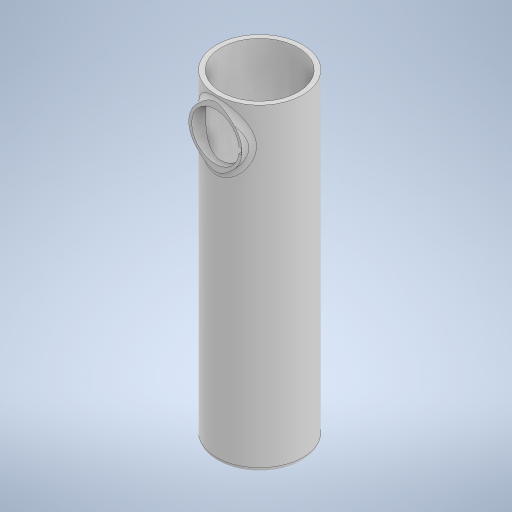
# Autodesk Inventor part: Flash_light
Saved by Autodesk Inventor 2024.2 (Build 282272000, 272)
## iProperties
Created: 2025-04-08
Part Number: Flash_light
Material: Generic
Document SubType Name: Modeling
Designer: Svend
Density: 1 g/cm^3
Appearance: Default
Author: Svend
Autodesk Inventor part; units mm, degrees
ref_plane "YZ Plane" through (0, 0, 0) normal (1, 0, 0) x (0, 1, 0)
sketch "Sketch1" plane through (0, 0, 0) normal (0, 1, 0) x (-1, 0, 0)
  circle A0 centre (0, 0) radius 15
  circle A1 centre (0, 0) radius 18.2
  dimension "d0" = 30
  dimension "d1" = 36.4
  constraints: 2 centre point, 2 coincident
  measures "d0" diameter of A0
  measures "d1" diameter of A1
extrude "Extrusion1" add sketch "Sketch1" along normal blind 4 contours A0 | A1
sketch "Sketch2" plane through (0, 4, 0) normal (0, -1, 0) x (1, 0, 0)
  circle A0 centre (0, 0) radius 18.2 projected
  circle A1 centre (0, 0) radius 16.2
  dimension "d17" = 2
  constraints: 1 centre point
  measures "d17" radial gap between concentric circles of A0 A1
extrude "Extrusion2" add sketch "Sketch2" against normal blind 130
ref_plane "Work Plane1" through (0, 0, 18.6) normal (0, 0, 1) x (1, 0, 0)
ref_plane "Work Plane2" through (0, 0, 18.2) normal (0, 0, 1) x (1, 0, 0)
sketch "Sketch3" plane through (0, 0, 18.6) normal (0, 0, 1) x (1, 0, 0)
  line L0 (0, 134) -> (0, 119) construction
  circle A0 centre (0, 119) radius 10
  circle A1 centre (0, 119) radius 11.2
  line L1 (11, 120.2) -> (9.9277, 120.2)
  line L2 (9, 120.2) -> (9, 117.8) construction
  line L3 (9, 117.8) -> (9.9277, 117.8) construction
  line L4 (11, 117.8) -> (11, 120.2)
  line L5 (11, 120.2) -> (9, 117.8) construction
  line L6 (9, 120.2) -> (11, 117.8) construction
  line L7 (9.9277, 120.2) -> (9, 120.2) construction
  line L8 (9.9277, 117.8) -> (11, 117.8)
  line L9 (18.2, 134) -> (-18.2, 134) projected
  line L10 (0, 134) -> (0, 119) construction
  point P0 (0, 0)
  point P1 (10, 119)
  dimension "d9" = 20
  dimension "d19" = 1.2
  dimension "d29" = 1
  dimension "d30" = 2.4
  dimension "d31" = 15
  constraints: 20 end point, 5 parallel, 3 midpoint, 3 point on circle, 2 centre point, 2 horizontal, 2 perpendicular, 2 vertical, 1 coincident, 1 horizontal alignment, 1 vertical alignment
  measures "d9" diameter of A0
  measures "d19" radial gap between concentric circles of A1 A0
  measures "d29" distance from line of L4 A0.start
  measures "d30" distance of L4.start L1.start
  measures "d31" distance of L10.start L0.end
extrude "Extrusion4" add sketch "Sketch3" against normal up to surface contours A0 | A0 L1 L4 L8 | A1 round surface about axis through (0, 0, 0) along (0, 1, 0) radius 18.2 far side no
extrude "Extrusion3" cut sketch "Sketch3" against normal blind 10 contours A0 | A0 L1 L4 L8
fillet "Fillet1" radius 3 3 edges at (8.5118, 111.7206, 16.0869) (8.5097, 126.2819, 16.0881) (-11.2, 118.9944, 14.3457)
fillet "Fillet2" radius 2 1 edges at (18.2, 0, 0)
ref_plane "Work Plane3" through (0, 0, 17.6) normal (0, 0, 1) x (1, 0, 0)
sketch "Sketch4" plane through (0, 0, 17.6) normal (0, 0, 1) x (1, 0, 0)
  line L0 (-4.6347, 132.1337) -> (-4.6347, 134) projected
  line L1 (-4.6347, 134) -> (4.6347, 134) projected
  line L2 (4.6347, 134) -> (4.6347, 132.1337) projected
  arc A0 (9.3217, 112.7915) -> (9.3217, 125.2085) centre (0, 119) ccw projected
  line L3 (4.6347, 105.8663) -> (4.6347, 2) projected
  line L4 (-4.6347, 2) -> (-4.6347, 105.8663) projected
  arc A1 (-9.3217, 125.2085) -> (-9.3217, 112.7915) centre (0, 119) ccw projected
  line L5 (0, 89) -> (-10, 89) construction
  line L6 (0, 89) -> (10, 89) construction
  line L7 (-2.5, 78) -> (2.5, 78)
  line L8 (2.5, 78) -> (2.5, 100)
  line L9 (2.5, 100) -> (-2.5, 100)
  line L10 (-2.5, 100) -> (-2.5, 78)
  line L11 (-2.5, 78) -> (2.5, 100) construction
  line L12 (2.5, 78) -> (-2.5, 100) construction
  line L13 (11, 120.2) -> (9.9277, 120.2) projected
  arc A2 (9.9277, 120.2) -> (9.9277, 117.8) centre (0, 119) ccw projected
  line L14 (9.9277, 117.8) -> (11, 117.8) projected
  line L15 (11, 117.8) -> (11, 120.2) projected
  point P0 (0, 0)
  dimension "d24" = 5
  dimension "d25" = 22
  constraints: 16 end point, 2 horizontal, 2 midpoint, 2 parallel, 1 horizontal alignment, 1 perpendicular, 1 point on line, 4 other
  measures "d24" distance of L9.end L8.end
  measures "d25" distance of L8.end L7.end
extrude "Extrusion5" cut sketch "Sketch4" against normal up to surface contours L10 L9 L8 L7 round surface about axis through (0, 4, 0) along (0, 1, 0) radius 16.2 far side no
body "Solid1"
